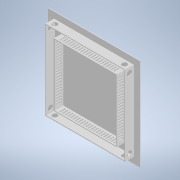
# Autodesk Inventor part: middle
Saved by Autodesk Inventor 2020 (Build 240168000, 168)
## iProperties
Created: 2020-05-02
Part Number: middle
Material: Generic
Document SubType Name: Modeling
Designer: galaxy
Density: 1 g/cm^3
Appearance: Default
Author: galaxy
Autodesk Inventor part; units mm, degrees
ref_plane "YZ Plane" through (0, 0, 0) normal (1, 0, 0) x (0, 1, 0)
ref_plane "XZ Plane" through (0, 0, 0) normal (0, 1, 0) x (-1, 0, 0)
ref_plane "XY Plane" through (0, 0, 0) normal (0, 0, 1) x (1, 0, 0)
sketch "Sketch1" plane through (0, 0, 0) normal (0, 0, 1) x (1, 0, 0)
  line L0 (-180, 180) -> (180, 180)
  line L1 (180, 180) -> (180, -180)
  line L2 (180, -180) -> (-180, -180)
  line L3 (-180, -180) -> (-180, 180)
  line L4 (-180, 180) -> (180, -180) construction
  line L5 (180, 180) -> (-180, -180) construction
  line L6 (-100, 100) -> (100, -100) construction
  line L7 (100, 100) -> (-100, -100) construction
  line L8 (-120, 120) -> (120, 120)
  line L9 (120, 120) -> (120, -120)
  line L10 (120, -120) -> (-120, -120)
  line L11 (-120, -120) -> (-120, 120)
  line L12 (-120, 120) -> (120, -120) construction
  line L13 (120, 120) -> (-120, -120) construction
  line L14 (-123, 123) -> (123, 123)
  line L15 (123, 123) -> (123, -123)
  line L16 (123, -123) -> (-123, -123)
  line L17 (-123, -123) -> (-123, 123)
  line L18 (-123, 123) -> (123, -123) construction
  line L19 (123, 123) -> (-123, -123) construction
  line L20 (-153, 153) -> (153, 153)
  line L21 (153, 153) -> (153, -153)
  line L22 (153, -153) -> (-153, -153)
  line L23 (-153, -153) -> (-153, 153)
  line L24 (-153, 153) -> (153, -153) construction
  line L25 (153, 153) -> (-153, -153) construction
  line L26 (-156, 156) -> (156, 156)
  line L27 (156, 156) -> (156, -156)
  line L28 (156, -156) -> (-156, -156)
  line L29 (-156, -156) -> (-156, 156)
  line L30 (-156, 156) -> (156, -156) construction
  line L31 (156, 156) -> (-156, -156) construction
  point P0 (0, 0)
  dimension "d0" = 360
  dimension "d1" = 360
  dimension "d4" = 240
  dimension "d5" = 240
  dimension "d6" = 246
  dimension "d7" = 246
  dimension "d8" = 306
  dimension "d9" = 306
  dimension "d10" = 312
  dimension "d11" = 312
  constraints: 64 end point, 12 midpoint, 10 parallel, 5 horizontal, 5 perpendicular
  measures "d0" distance of L1.end L2.end
  measures "d1" distance of L0.end L1.end
  measures "d4" distance of L9.end L10.end
  measures "d5" distance of L8.end L9.end
  measures "d6" distance of L15.end L16.end
  measures "d7" distance of L14.end L15.end
  measures "d8" distance of L21.end L22.end
  measures "d9" distance of L20.end L21.end
  measures "d10" distance of L27.end L28.end
  measures "d11" distance of L26.end L27.end
extrude "Extrusion2" add sketch "Sketch1" along normal blind 3 contours L8 L9 L10 L11
extrude "Extrusion3" add sketch "Sketch1" along normal blind 3 contours L20 L21 L22 L23
extrude "Extrusion4" add sketch "Sketch1" along normal blind 3 contours L0 L1 L2 L3
extrude "Extrusion5" add sketch "Sketch1" along normal blind 37 contours L26 L27 L28 L29
extrude "Extrusion6" add sketch "Sketch1" along normal blind 37 contours L14 L15 L16 L17
sketch "Sketch2" plane through (-120, -120, 3) normal (0, 1, 0) x (1, 0, 0)
  line L0 (12.5, -8) -> (17.5, -8)
  line L1 (17.5, -8) -> (17.5, -29)
  line L2 (17.5, -29) -> (12.5, -29)
  line L3 (12.5, -29) -> (12.5, -8)
  line L4 (12.5, -8) -> (17.5, -29) construction
  line L5 (17.5, -8) -> (12.5, -29) construction
  line L6 (0, 0) -> (240, 0) projected
  line L7 (22.5, -8) -> (27.5, -8)
  line L8 (27.5, -8) -> (27.5, -29)
  line L9 (27.5, -29) -> (22.5, -29)
  line L10 (22.5, -29) -> (22.5, -8)
  line L11 (22.5, -8) -> (27.5, -29) construction
  line L12 (27.5, -8) -> (22.5, -29) construction
  line L13 (32.5, -8) -> (37.5, -8)
  line L14 (37.5, -8) -> (37.5, -29)
  line L15 (37.5, -29) -> (32.5, -29)
  line L16 (32.5, -29) -> (32.5, -8)
  line L17 (32.5, -8) -> (37.5, -29) construction
  line L18 (37.5, -8) -> (32.5, -29) construction
  line L19 (42.5, -8) -> (47.5, -8)
  line L20 (47.5, -8) -> (47.5, -29)
  line L21 (47.5, -29) -> (42.5, -29)
  line L22 (42.5, -29) -> (42.5, -8)
  line L23 (42.5, -8) -> (47.5, -29) construction
  line L24 (47.5, -8) -> (42.5, -29) construction
  line L25 (52.5, -8) -> (57.5, -8)
  line L26 (57.5, -8) -> (57.5, -29)
  line L27 (57.5, -29) -> (52.5, -29)
  line L28 (52.5, -29) -> (52.5, -8)
  line L29 (52.5, -8) -> (57.5, -29) construction
  line L30 (57.5, -8) -> (52.5, -29) construction
  line L31 (62.5, -8) -> (67.5, -8)
  line L32 (67.5, -8) -> (67.5, -29)
  line L33 (67.5, -29) -> (62.5, -29)
  line L34 (62.5, -29) -> (62.5, -8)
  line L35 (62.5, -8) -> (67.5, -29) construction
  line L36 (67.5, -8) -> (62.5, -29) construction
  line L37 (72.5, -8) -> (77.5, -8)
  line L38 (77.5, -8) -> (77.5, -29)
  line L39 (77.5, -29) -> (72.5, -29)
  line L40 (72.5, -29) -> (72.5, -8)
  line L41 (72.5, -8) -> (77.5, -29) construction
  line L42 (77.5, -8) -> (72.5, -29) construction
  line L43 (82.5, -8) -> (87.5, -8)
  line L44 (87.5, -8) -> (87.5, -29)
  line L45 (87.5, -29) -> (82.5, -29)
  line L46 (82.5, -29) -> (82.5, -8)
  line L47 (92.5, -8) -> (97.5, -8)
  line L48 (97.5, -8) -> (97.5, -29)
  line L49 (97.5, -29) -> (92.5, -29)
  line L50 (92.5, -29) -> (92.5, -8)
  line L51 (102.5, -8) -> (107.5, -8)
  line L52 (107.5, -8) -> (107.5, -29)
  line L53 (107.5, -29) -> (102.5, -29)
  line L54 (102.5, -29) -> (102.5, -8)
  line L55 (112.5, -8) -> (117.5, -8)
  line L56 (117.5, -8) -> (117.5, -29)
  line L57 (117.5, -29) -> (112.5, -29)
  line L58 (112.5, -29) -> (112.5, -8)
  line L59 (122.5, -8) -> (127.5, -8)
  line L60 (127.5, -8) -> (127.5, -29)
  line L61 (127.5, -29) -> (122.5, -29)
  line L62 (122.5, -29) -> (122.5, -8)
  line L63 (132.5, -8) -> (137.5, -8)
  line L64 (137.5, -8) -> (137.5, -29)
  line L65 (137.5, -29) -> (132.5, -29)
  line L66 (132.5, -29) -> (132.5, -8)
  line L67 (142.5, -8) -> (147.5, -8)
  line L68 (147.5, -8) -> (147.5, -29)
  line L69 (147.5, -29) -> (142.5, -29)
  line L70 (142.5, -29) -> (142.5, -8)
  line L71 (152.5, -8) -> (157.5, -8)
  line L72 (157.5, -8) -> (157.5, -29)
  line L73 (157.5, -29) -> (152.5, -29)
  line L74 (152.5, -29) -> (152.5, -8)
  line L75 (152.5, -8) -> (157.5, -29) construction
  line L76 (157.5, -8) -> (152.5, -29) construction
  line L77 (162.5, -8) -> (167.5, -8)
  line L78 (167.5, -8) -> (167.5, -29)
  line L79 (167.5, -29) -> (162.5, -29)
  line L80 (162.5, -29) -> (162.5, -8)
  line L81 (172.5, -8) -> (177.5, -8)
  line L82 (177.5, -8) -> (177.5, -29)
  line L83 (177.5, -29) -> (172.5, -29)
  line L84 (172.5, -29) -> (172.5, -8)
  line L85 (182.5, -8) -> (187.5, -8)
  line L86 (187.5, -8) -> (187.5, -29)
  line L87 (187.5, -29) -> (182.5, -29)
  line L88 (192.5, -8) -> (197.5, -8)
  line L89 (197.5, -8) -> (197.5, -29)
  line L90 (197.5, -29) -> (192.5, -29)
  line L91 (182.05, -29) -> (182.05, -8)
  line L92 (182.05, -8) -> (187.05, -8)
  line L93 (187.05, -29) -> (182.05, -29)
  line L94 (192.05, -29) -> (192.05, -8)
  line L95 (192.05, -8) -> (197.05, -8)
  line L96 (197.05, -29) -> (192.05, -29)
  line L97 (202.5, -29) -> (202.5, -8)
  line L98 (202.5, -8) -> (207.5, -8)
  line L99 (207.5, -8) -> (202.5, -29) construction
  line L100 (202.5, -8) -> (207.5, -29) construction
  line L101 (207.5, -29) -> (202.5, -29)
  line L102 (207.5, -8) -> (207.5, -29)
  line L103 (212.5, -29) -> (212.5, -8)
  line L104 (217.5, -8) -> (212.5, -29) construction
  line L105 (217.5, -8) -> (217.5, -29)
  line L106 (212.5, -8) -> (217.5, -29) construction
  line L107 (212.5, -8) -> (217.5, -8)
  line L108 (222.5, -29) -> (222.5, -8)
  line L109 (222.5, -8) -> (227.5, -8)
  line L110 (227.5, -8) -> (222.5, -29) construction
  line L111 (222.5, -8) -> (227.5, -29) construction
  line L112 (227.5, -29) -> (222.5, -29)
  line L113 (227.5, -8) -> (227.5, -29)
  line L114 (217.5, -29) -> (212.5, -29)
  point P0 (120, 3)
  point P1 (15, -18.5)
  point P2 (0, -34)
  point P3 (25, -18.5)
  point P4 (35, -18.5)
  point P5 (45, -18.5)
  point P6 (55, -18.5)
  point P7 (65, -18.5)
  point P8 (75, -18.5)
  point P9 (155, -18.5)
  point P10 (205, -18.5)
  point P11 (215, -18.5)
  point P12 (225, -18.5)
  point P13 (192.5, -29)
  dimension "d24" = 5
  dimension "d25" = 21
  dimension "d26" = 12.5
  dimension "d27" = 8
  dimension "d30" = 5
  dimension "d31" = 21
  dimension "d32" = 5
  dimension "d33" = 21
  dimension "d34" = 5
  dimension "d35" = 21
  dimension "d36" = 5
  dimension "d37" = 21
  dimension "d38" = 5
  dimension "d39" = 21
  dimension "d40" = 5
  dimension "d42" = 5
  dimension "d44" = 5
  dimension "d46" = 5
  dimension "d48" = 5
  dimension "d50" = 5
  dimension "d52" = 5
  dimension "d53" = 21
  dimension "d54" = 8
  dimension "d55" = 8
  dimension "d56" = 8
  dimension "d66" = 5
  dimension "d67" = 5
  dimension "d68" = 5
  dimension "d69" = 5
  dimension "d70" = 5
  dimension "d71" = 5
  dimension "d72" = 5
  dimension "d73" = 5
  dimension "d74" = 5
  dimension "d75" = 5
  dimension "d76" = 5
  dimension "d77" = 5
  dimension "d95" = 5
  dimension "d96" = 21
  dimension "d97" = 5
  dimension "d99" = 5
  dimension "d101" = 5
  dimension "d103" = 5
  dimension "d105" = 5
  dimension "d106" = 21
  dimension "d107" = 5
  dimension "d108" = 5
  dimension "d109" = 5
  dimension "d112" = 5
  dimension "d117" = 5
  dimension "d119" = 5
  dimension "d120" = 21
  dimension "d124" = 5
  dimension "d125" = 21
  dimension "d126" = 5
  dimension "d127" = 21
  dimension "d128" = 5
  dimension "d132" = 5
  dimension "d133" = 5
  dimension "d135" = 8
  dimension "d136" = 5
  constraints: 228 end point, 44 parallel, 24 horizontal, 22 midpoint, 22 perpendicular
  measures "d24" distance of L1.end L2.end
  measures "d25" distance of L0.end L1.end
  measures "d26" distance from line of point (0, -34) L3
  measures "d27" distance between parallel lines of L6 L0
  measures "d30" distance of L8.end L9.end
  measures "d31" distance of L7.end L8.end
  measures "d32" distance of L14.end L15.end
  measures "d33" distance of L13.end L14.end
  measures "d34" distance of L20.end L21.end
  measures "d35" distance of L19.end L20.end
  measures "d36" distance of L26.end L27.end
  measures "d37" distance of L25.end L26.end
  measures "d38" distance of L32.end L33.end
  measures "d39" distance of L31.end L32.end
  measures "d40" distance of L38.end L39.end
  measures "d42" distance of L44.end L45.end
  measures "d44" distance of L48.end L49.end
  measures "d46" distance of L52.end L53.end
  measures "d48" distance of L56.end L57.end
  measures "d50" distance of L60.end L61.end
  measures "d52" distance of L64.end L65.end
  measures "d53" distance of L63.end L64.end
  measures "d54" distance between parallel lines of L6 L7
  measures "d55" distance between parallel lines of L6 L13
  measures "d56" distance between parallel lines of L6 L19
  measures "d66" distance between parallel lines of L1 L10
  measures "d67" distance between parallel lines of L16 L8
  measures "d68" distance between parallel lines of L22 L14
  measures "d69" distance between parallel lines of L28 L20
  measures "d70" distance between parallel lines of L34 L26
  measures "d71" distance between parallel lines of L40 L32
  measures "d72" distance between parallel lines of L38 L46
  measures "d73" distance between parallel lines of L50 L44
  measures "d74" distance between parallel lines of L54 L48
  measures "d75" distance between parallel lines of L58 L52
  measures "d76" distance between parallel lines of L62 L56
  measures "d77" distance between parallel lines of L66 L60
  measures "d95" distance of L68.end L70.start
  measures "d96" distance of L67.end L68.end
  measures "d97" distance of L73.start L74.start
  measures "d99" distance of L79.start L79.end
  measures "d101" distance of L82.end L84.start
  measures "d103" distance of L87.start L87.end
  measures "d105" distance of L89.end L90.end
  measures "d106" distance of L88.end L89.end
  measures "d107" distance between parallel lines of L74 L68
  measures "d108" distance between parallel lines of L80 L72
  measures "d109" distance between parallel lines of L84 L78
  measures "d112" distance between parallel lines of L64 L70
  measures "d117" distance of L93.start L91.start
  measures "d119" distance of L96.start L94.start
  measures "d120" distance of L95.end L96.start
  measures "d124" distance of L101.start L97.start
  measures "d125" distance of L98.end L101.start
  measures "d126" distance of L105.end L103.start
  measures "d127" distance of L105.start L105.end
  measures "d128" distance of L112.start L108.start
  measures "d132" distance between parallel lines of L103 L102
  measures "d133" distance between parallel lines of L108 L105
  measures "d135" distance between parallel lines of L6 L98
  measures "d136" distance between parallel lines of L89 L97
extrude "Extrusion7" cut sketch "Sketch2" against normal blind 3 contours L0 L1 L2 L3
extrude "Extrusion8" cut sketch "Sketch2" against normal blind 3 contours L7 L8 L9 L10
extrude "Extrusion9" cut sketch "Sketch2" against normal blind 3 contours L13 L14 L15 L16
extrude "Extrusion10" cut sketch "Sketch2" against normal blind 3 contours L19 L20 L21 L22
extrude "Extrusion11" cut sketch "Sketch2" against normal blind 3 contours L25 L26 L27 L28
extrude "Extrusion12" cut sketch "Sketch2" against normal blind 3 contours L31 L32 L33 L34
extrude "Extrusion13" cut sketch "Sketch2" against normal blind 3 contours L37 L38 L39 L40
extrude "Extrusion14" cut sketch "Sketch2" against normal blind 3 contours L108 L109 L113 L112
extrude "Extrusion15" cut sketch "Sketch2" against normal blind 3 contours L103 L107 L105 L114
extrude "Extrusion16" cut sketch "Sketch2" against normal blind 3 contours L97 L98 L102 L101
extrude "Extrusion17" cut sketch "Sketch2" against normal blind 3 contours L71 L72 L73 L74
extrude "Extrusion18" cut sketch "Sketch2" against normal blind 3 contours L67 L68 L69 L70
extrude "Extrusion19" cut sketch "Sketch2" against normal blind 3 contours L88 L89 L90 L96 L94 L95
extrude "Extrusion20" cut sketch "Sketch2" against normal blind 3 contours L85 L86 L87 L93 L91 L92
extrude "Extrusion21" cut sketch "Sketch2" against normal blind 3 contours L81 L82 L83 L84
extrude "Extrusion22" cut sketch "Sketch2" against normal blind 3 contours L77 L78 L79 L80
extrude "Extrusion23" cut sketch "Sketch2" against normal blind 3 contours L63 L64 L65 L66
extrude "Extrusion24" cut sketch "Sketch2" against normal blind 3 contours L59 L60 L61 L62
extrude "Extrusion25" cut sketch "Sketch2" against normal blind 3 contours L43 L44 L45 L46
extrude "Extrusion26" cut sketch "Sketch2" against normal blind 3 contours L47 L48 L49 L50
extrude "Extrusion27" cut sketch "Sketch2" against normal blind 3 contours L51 L52 L53 L54
extrude "Extrusion28" cut sketch "Sketch2" against normal blind 3 contours L55 L56 L57 L58
mirror "Mirror1" about plane through (0, 0, 0) normal (0, 1, 0) of "Extrusion7", "Extrusion8", "Extrusion9", "Extrusion10", "Extrusion11", "Extrusion12"
mirror "Mirror2" about plane through (0, 0, 0) normal (0, 1, 0) of "Extrusion13", "Extrusion25", "Extrusion26", "Extrusion27", "Extrusion28", "Extrusion24", "Extrusion23", "Extrusion18", "Extrusion17", "Extrusion22", "Extrusion21", "Extrusion20", "Extrusion19", "Extrusion16", "Extrusion15", "Extrusion14"
sketch "Sketch4" plane through (120, -120, 3) normal (-1, 0, 0) x (0, 0, 1)
  line L0 (8, 12.5) -> (29, 12.5)
  line L1 (29, 12.5) -> (29, 17.5)
  line L2 (29, 17.5) -> (8, 17.5)
  line L3 (8, 17.5) -> (8, 12.5)
  line L4 (8, 12.5) -> (29, 17.5) construction
  line L5 (29, 12.5) -> (8, 17.5) construction
  line L6 (0, 0) -> (0, 240) projected
  line L7 (8, 22.5) -> (29, 22.5)
  line L8 (29, 22.5) -> (29, 27.5)
  line L9 (29, 27.5) -> (8, 27.5)
  line L10 (8, 27.5) -> (8, 22.5)
  line L11 (8, 22.5) -> (29, 27.5) construction
  line L12 (29, 22.5) -> (8, 27.5) construction
  line L13 (8, 32.5) -> (29, 32.5)
  line L14 (29, 32.5) -> (29, 37.5)
  line L15 (29, 37.5) -> (8, 37.5)
  line L16 (8, 37.5) -> (8, 32.5)
  line L17 (8, 32.5) -> (29, 37.5) construction
  line L18 (29, 32.5) -> (8, 37.5) construction
  line L19 (8, 42.5) -> (29, 42.5)
  line L20 (29, 42.5) -> (29, 47.5)
  line L21 (29, 47.5) -> (8, 47.5)
  line L22 (8, 47.5) -> (8, 42.5)
  line L23 (8, 42.5) -> (29, 47.5) construction
  line L24 (29, 42.5) -> (8, 47.5) construction
  line L25 (8, 52.5) -> (29, 52.5)
  line L26 (29, 52.5) -> (29, 57.5)
  line L27 (29, 57.5) -> (8, 57.5)
  line L28 (8, 57.5) -> (8, 52.5)
  line L29 (8, 52.5) -> (29, 57.5) construction
  line L30 (29, 52.5) -> (8, 57.5) construction
  line L31 (8, 62.5) -> (29, 62.5)
  line L32 (29, 62.5) -> (29, 67.5)
  line L33 (29, 67.5) -> (8, 67.5)
  line L34 (8, 67.5) -> (8, 62.5)
  line L35 (8, 62.5) -> (29, 67.5) construction
  line L36 (29, 62.5) -> (8, 67.5) construction
  line L37 (8, 72.5) -> (29, 72.5)
  line L38 (29, 72.5) -> (29, 77.5)
  line L39 (29, 77.5) -> (8, 77.5)
  line L40 (8, 77.5) -> (8, 72.5)
  line L41 (8, 72.5) -> (29, 77.5) construction
  line L42 (29, 72.5) -> (8, 77.5) construction
  line L43 (8, 82.5) -> (29, 82.5)
  line L44 (29, 82.5) -> (29, 87.5)
  line L45 (29, 87.5) -> (8, 87.5)
  line L46 (8, 87.5) -> (8, 82.5)
  line L47 (8, 82.5) -> (29, 87.5) construction
  line L48 (29, 82.5) -> (8, 87.5) construction
  line L49 (8, 92.5) -> (29, 92.5)
  line L50 (29, 92.5) -> (29, 97.5)
  line L51 (29, 97.5) -> (8, 97.5)
  line L52 (8, 97.5) -> (8, 92.5)
  line L53 (8, 92.5) -> (29, 97.5) construction
  line L54 (29, 92.5) -> (8, 97.5) construction
  line L55 (8, 102.5) -> (29, 102.5)
  line L56 (29, 102.5) -> (29, 107.5)
  line L57 (29, 107.5) -> (8, 107.5)
  line L58 (8, 107.5) -> (8, 102.5)
  line L59 (8, 102.5) -> (29, 107.5) construction
  line L60 (29, 102.5) -> (8, 107.5) construction
  line L61 (8, 112.5) -> (29, 112.5)
  line L62 (29, 112.5) -> (29, 117.5)
  line L63 (29, 117.5) -> (8, 117.5)
  line L64 (8, 117.5) -> (8, 112.5)
  line L65 (8, 112.5) -> (29, 117.5) construction
  line L66 (29, 112.5) -> (8, 117.5) construction
  line L67 (8, 122.5) -> (29, 122.5)
  line L68 (29, 122.5) -> (29, 127.5)
  line L69 (29, 127.5) -> (8, 127.5)
  line L70 (8, 127.5) -> (8, 122.5)
  line L71 (8, 122.5) -> (29, 127.5) construction
  line L72 (29, 122.5) -> (8, 127.5) construction
  line L73 (8, 132.5) -> (29, 132.5)
  line L74 (29, 132.5) -> (29, 137.5)
  line L75 (29, 137.5) -> (8, 137.5)
  line L76 (8, 137.5) -> (8, 132.5)
  line L77 (8, 132.5) -> (29, 137.5) construction
  line L78 (29, 132.5) -> (8, 137.5) construction
  line L79 (8, 142.5) -> (29, 142.5)
  line L80 (29, 142.5) -> (29, 147.5)
  line L81 (29, 147.5) -> (8, 147.5)
  line L82 (8, 147.5) -> (8, 142.5)
  line L83 (8, 142.5) -> (29, 147.5) construction
  line L84 (29, 142.5) -> (8, 147.5) construction
  line L85 (8, 152.5) -> (29, 152.5)
  line L86 (29, 152.5) -> (29, 157.5)
  line L87 (29, 157.5) -> (8, 157.5)
  line L88 (8, 157.5) -> (8, 152.5)
  line L89 (8, 152.5) -> (29, 157.5) construction
  line L90 (29, 152.5) -> (8, 157.5) construction
  line L91 (8, 162.5) -> (29, 162.5)
  line L92 (29, 162.5) -> (29, 167.5)
  line L93 (29, 167.5) -> (8, 167.5)
  line L94 (8, 167.5) -> (8, 162.5)
  line L95 (8, 162.5) -> (29, 167.5) construction
  line L96 (29, 162.5) -> (8, 167.5) construction
  line L97 (8, 172.5) -> (29, 172.5)
  line L98 (29, 172.5) -> (29, 177.5)
  line L99 (29, 177.5) -> (8, 177.5)
  line L100 (8, 177.5) -> (8, 172.5)
  line L101 (8, 172.5) -> (29, 177.5) construction
  line L102 (29, 172.5) -> (8, 177.5) construction
  line L103 (8, 182.5) -> (29, 182.5)
  line L104 (29, 182.5) -> (29, 187.5)
  line L105 (29, 187.5) -> (8, 187.5)
  line L106 (8, 187.5) -> (8, 182.5)
  line L107 (8, 182.5) -> (29, 187.5) construction
  line L108 (29, 182.5) -> (8, 187.5) construction
  line L109 (8, 192.5) -> (29, 192.5)
  line L110 (29, 192.5) -> (29, 197.5)
  line L111 (29, 197.5) -> (8, 197.5)
  line L112 (8, 197.5) -> (8, 192.5)
  line L113 (8, 192.5) -> (29, 197.5) construction
  line L114 (29, 192.5) -> (8, 197.5) construction
  line L115 (8, 202.5) -> (29, 202.5)
  line L116 (29, 202.5) -> (29, 207.5)
  line L117 (29, 207.5) -> (8, 207.5)
  line L118 (8, 207.5) -> (8, 202.5)
  line L119 (8, 202.5) -> (29, 207.5) construction
  line L120 (29, 202.5) -> (8, 207.5) construction
  line L121 (8, 212.5) -> (29, 212.5)
  line L122 (29, 212.5) -> (29, 217.5)
  line L123 (29, 217.5) -> (8, 217.5)
  line L124 (8, 217.5) -> (8, 212.5)
  line L125 (8, 212.5) -> (29, 217.5) construction
  line L126 (29, 212.5) -> (8, 217.5) construction
  line L127 (8, 222.5) -> (29, 222.5)
  line L128 (29, 222.5) -> (29, 227.5)
  line L129 (29, 227.5) -> (8, 227.5)
  line L130 (8, 227.5) -> (8, 222.5)
  line L131 (8, 222.5) -> (29, 227.5) construction
  line L132 (29, 222.5) -> (8, 227.5) construction
  point P0 (-3, 120)
  point P1 (18.5, 15)
  point P2 (34, 0)
  point P3 (18.5, 25)
  point P4 (18.5, 35)
  point P5 (18.5, 45)
  point P6 (18.5, 55)
  point P7 (18.5, 65)
  point P8 (18.5, 75)
  point P9 (18.5, 85)
  point P10 (18.5, 95)
  point P11 (18.5, 105)
  point P12 (18.5, 115)
  point P13 (18.5, 125)
  point P14 (18.5, 135)
  point P15 (18.5, 145)
  point P16 (18.5, 155)
  point P17 (18.5, 165)
  point P18 (18.5, 175)
  point P19 (18.5, 185)
  point P20 (18.5, 195)
  point P21 (18.5, 205)
  point P22 (18.5, 215)
  point P23 (18.5, 225)
  dimension "d181" = 21
  dimension "d182" = 5
  dimension "d183" = 12.5
  dimension "d184" = 8
  dimension "d187" = 10
  constraints: 264 end point, 44 midpoint, 2 parallel, 1 horizontal, 1 perpendicular, 1 vertical, 231 other
  measures "d181" distance of L2.end L1.end
  measures "d182" distance of L1.end L0.end
  measures "d183" distance from line of point (34, 0) L0
  measures "d184" distance between parallel lines of L6 L3
  measures "d187" distance of L0.start L7.start
extrude "Extrusion29" cut sketch "Sketch4" against normal blind 3 contours L16 L15 L14 L13 | L22 L21 L20 L19 | L28 L27 L26 L25 | L34 L33 L32 L31 | L40 L39 L38 L37 | L46 L45 L44 L43 | L52 L51 L50 L49 | L58 L57 L56 L55 | L64 L63 L62 L61 | L70 L69 L68 L67 | L76 L75 L74 L73 | L82 L81 L80 L79 | L88 L87 L86 L85 | L94 L93 L92 L91 | L100 L99 L98 L97 | L106 L105 L104 L103 | L112 L111 L110 L109 | L118 L117 L116 L115 | L124 L123 L122 L121 | L130 L129 L128 L127
extrude "Extrusion30" cut sketch "Sketch4" against normal blind 3 contours L10 L9 L8 L7
extrude "Extrusion31" cut sketch "Sketch4" against normal blind 3 contours L3 L2 L1 L0
mirror "Mirror3" about plane through (0, 0, 0) normal (1, 0, 0) of "Extrusion29", "Extrusion30", "Extrusion31"
sketch "Sketch5" plane through (-156, 156, 3) normal (0, 1, 0) x (1, 0, 0)
  circle A0 centre (20, -17) radius 10
  line L0 (0, 0) -> (0, -34) projected
  line L1 (336, 0) -> (-24, 0) projected
  circle A1 centre (292, -17) radius 10
  line L2 (312, 0) -> (312, -34) projected
  point P0 (156, 3)
  dimension "d198" = 20
  dimension "d199" = 20
  dimension "d200" = 17
  dimension "d201" = 20
  dimension "d202" = 20
  dimension "d203" = 17
  constraints: 2 centre point
  measures "d198" diameter of A0
  measures "d199" distance from line of L0 A0.centre
  measures "d200" distance from line of L1 A0.centre
  measures "d201" diameter of A1
  measures "d202" distance from line of L2 A1.centre
  measures "d203" distance from line of L1 A1.centre
extrude "Extrusion32" cut sketch "Sketch5" against normal blind 3
mirror "Mirror4" about plane through (0, 0, 0) normal (0, 1, 0) of "Extrusion32"
sketch "Sketch6" plane through (156, -156, 3) normal (1, 0, 0) x (0, 0, -1)
  circle A0 centre (-17, 292) radius 10
  line L0 (0, 312) -> (-34, 312) projected
  line L1 (-34, 0) -> (-34, 312) projected
  line L2 (-34, 3) -> (-34, 309) projected
  line L3 (-34, 156) -> (3, 156)
  circle A1 centre (-17, 20) radius 10
  dimension "d206" = 20
  dimension "d207" = 20
  dimension "d208" = 17
  constraints: 2 centre point, 2 end point, 1 horizontal, 1 midpoint, 1 symmetric about line, 1 other
  measures "d206" diameter of A0
  measures "d207" distance from line of L0 A0.centre
  measures "d208" distance from line of L1 A0.centre
extrude "Extrusion33" cut sketch "Sketch6" against normal blind 3
mirror "Mirror5" about plane through (0, 0, 0) normal (1, 0, 0) of "Extrusion33"
sketch "Sketch8" plane through (0, 0, 3) normal (0, 0, 1) x (1, 0, 0)
  circle A0 centre (-171, 148) radius 1.5
  circle A1 centre (-171, 134) radius 1.5
  line L0 (180, 180) -> (-180, 180) projected
  line L1 (-180, 180) -> (-180, -180) projected
  point P0 (0, 0)
  dimension "d219" = 3
  dimension "d220" = 3
  dimension "d223" = 32
  dimension "d224" = 14
  dimension "d225" = 9
  dimension "d226" = 9
  constraints: 2 centre point
  measures "d219" diameter of A0
  measures "d220" diameter of A1
  measures "d223" distance from line of L0 A0.centre
  measures "d224" distance of A1.centre A0.centre
  measures "d225" distance from line of L1 A0.centre
  measures "d226" distance from line of L1 A1.centre
extrude "Extrusion35" cut sketch "Sketch8" against normal blind 10
body "Solid2"
